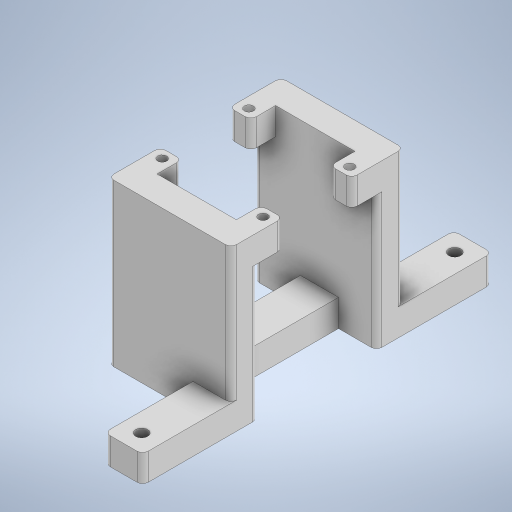
# Autodesk Inventor part: lepton mount
Saved by Autodesk Inventor 2024 (Build 280153000, 153)
## iProperties
Created: 2024-01-12
Part Number: lepton mount
Material: Generic
Document SubType Name: Modeling
Designer: Eli
Density: 1 g/cm^3
Appearance: Default
Author: Eli
Autodesk Inventor part; units mm, degrees
ref_plane "YZ Plane" through (0, 0, 0) normal (1, 0, 0) x (0, 1, 0)
ref_plane "XZ Plane" through (0, 0, 0) normal (0, 1, 0) x (-1, 0, 0)
ref_plane "XY Plane" through (0, 0, 0) normal (0, 0, 1) x (1, 0, 0)
sketch "Sketch1" plane through (0, 0, 0) normal (0, 1, 0) x (-1, 0, 0)
  line L0 (0, 0) -> (-8.9535, 0)
  line L1 (-8.9535, 0) -> (-8.9535, -82.296)
  line L2 (-8.9535, -82.296) -> (0, -82.296)
  line L3 (0, -82.296) -> (0, 0)
  circle A0 centre (-4.4767, -4.2545) radius 1.4224
  line L4 (0, -41.148) -> (-8.9535, -41.148) construction
  circle A1 centre (-4.4767, -78.0415) radius 1.4224
  line L5 (0, -20.828) -> (19.9009, -20.828)
  line L6 (19.9009, -20.828) -> (19.9009, -61.468)
  line L7 (19.9009, -61.468) -> (0, -61.468)
  line L8 (0, -61.468) -> (0, -20.828)
  line L9 (19.9009, -55.118) -> (0, -55.118)
  line L10 (0, -55.118) -> (0, -27.178)
  line L11 (0, -27.178) -> (19.9009, -27.178)
  line L12 (19.9009, -27.178) -> (19.9009, -55.118)
  line L13 (0, -55.118) -> (8.9662, -55.118)
  line L14 (8.9662, -55.118) -> (8.9662, -27.178)
  line L15 (8.9662, -27.178) -> (0, -27.178)
  line L16 (0, -27.178) -> (0, -55.118)
  line L17 (0, -27.178) -> (-8.9535, -27.178)
  line L18 (0, -55.118) -> (-8.9535, -55.118)
  line L19 (0, -20.828) -> (-8.9535, -20.828)
  line L20 (0, -61.468) -> (-8.9535, -61.468)
  point P0 (-4.4768, 0)
  point P1 (0, -61.468)
  point P2 (0, -55.118)
  point P3 (19.9009, -27.178)
  point P4 (0, -55.118)
  point P5 (0, -61.468)
  dimension "d0" = 82.296
  dimension "d1" = 8.9535
  dimension "d2" = 2.8448
  dimension "d3" = 4.2545
  dimension "d4" = 4.4768
  dimension "d5" = 40.64
  dimension "d6" = 19.9009
  dimension "d11" = 27.94
  dimension "d28" = 8.9662
  constraints: 42 end point, 8 parallel, 8 perpendicular, 8 point on line, 4 horizontal, 3 midpoint, 2 centre point, 1 symmetric about line, 3 other
  measures "d0" distance of L0.end L1.end
  measures "d1" distance of L0.start L0.end
  measures "d2" diameter of A0
  measures "d3" distance of point (-4.477, 0) A0.centre
  measures "d4" distance from line of L3 A0.centre
  measures "d5" distance of L5.end L6.end
  measures "d6" distance between parallel lines of L8 L6
  measures "d11" distance between parallel lines of L11 L9
  measures "d28" distance between parallel lines of L8 L14
extrude "Extrusion1" add sketch "Sketch1" along normal blind 6.35 contours L3 L19 L1 L0 | L11 L14 L9 L3 | L3 L2 L1 L20
fillet "Fillet1" radius 1.27 4 edges at (8.9535, 3.175, 0) (0, 3.175, 0) (8.9535, 3.175, -82.296) (0, 3.175, -82.296)
extrude "Extrusion2" add sketch "Sketch1" along normal blind 38.1 contours L5 L6 L11 L3 | L3 L17 L1 L19 | L9 L6 L7 L3 | L3 L20 L1 L18
sketch "Sketch2" plane through (-19.9009, 0, -55.118) normal (0, 0, 1) x (1, 0, 0)
  line L0 (0, 38.1) -> (19.9009, 38.1) projected
  line L1 (19.9009, 38.1) -> (23.7744, 38.1)
  line L2 (23.7744, 38.1) -> (23.7744, 31.75)
  line L3 (23.7744, 31.75) -> (28.8544, 31.75)
  line L4 (28.8544, 31.75) -> (28.8544, 38.1)
  line L5 (28.8544, 0) -> (28.8544, 38.1) projected
  line L6 (23.7744, 38.1) -> (28.8544, 38.1)
  line L7 (28.8544, 38.1) -> (28.8544, 31.75)
  point P0 (19.9009, 0)
  point P1 (14.8209, 38.1)
  dimension "d14" = 6.35
  dimension "d15" = 5.08
  constraints: 12 end point, 2 parallel, 2 perpendicular, 1 collinear, 1 horizontal
  measures "d14" distance of L1.end L2.end
  measures "d15" distance of L2.end L3.end
extrude "Extrusion3" add sketch "Sketch2" along normal blind 5.842
sketch "Sketch3" plane through (0, 38.1, 0) normal (0, 1, 0) x (1, 0, 0)
  line L0 (-19.9009, 55.118) -> (-8.9662, 55.118) construction
  line L1 (3.8735, 49.276) -> (8.9535, 49.276) construction
  line L2 (6.4135, 49.276) -> (6.4135, 55.118) construction
  line L3 (0, 55.118) -> (8.9535, 55.118) construction
  point P0 (0, 0)
  point P1 (6.4135, 51.3715)
  dimension "d34" = 2.0955
  dimension "d35" = 0
  constraints: 2 end point, 1 midpoint, 1 point on line, 1 vertical
  measures "d34" distance from line of L1 point (6.413, 51.371)
  measures "d35" distance from line of L2 point (6.413, 51.371)
hole "Hole1" at (6.4135, 38.1, -51.3715) direction (0, -1, 0) diameter 2.1463 depth 6.35 tip angle 118
ref_plane "Work Plane1" through (-5.4737, 0, -81.026) normal (1, 0, 0) x (0, 0, -1)
mirror "Mirror1" about plane through (-5.4737, 0, -81.026) normal (1, 0, 0) of "Extrusion3", "Hole1"
ref_plane "Work Plane2" through (-19.9009, 0, -41.148) normal (0, 0, 1) x (1, 0, 0)
mirror "Mirror2" about plane through (-19.9009, 0, -41.148) normal (0, 0, 1) of "Extrusion3", "Hole1", "Mirror1"
fillet "Fillet2" radius 1.27 2 edges at (-19.9009, 19.05, -20.828) (-19.9009, 19.05, -61.468)
fillet "Fillet3" radius 1.27 8 edges at (8.9535, 34.925, -49.276) (3.8735, 34.925, -49.276) (-14.8209, 34.925, -49.276) (-19.9009, 34.925, -49.276) (-19.9009, 34.925, -33.02) (3.8735, 34.925, -33.02) (-14.8209, 34.925, -33.02) (8.9535, 34.925, -33.02)
fillet "Fillet5" radius 1.27 2 edges at (-19.9009, 15.875, -55.118) (-19.9009, 15.875, -27.178)
fillet "Fillet7" radius 1.27 2 edges at (8.9535, 15.875, -27.178) (8.9535, 15.875, -55.118)
fillet "Fillet10" radius 1.27 2 edges at (8.9535, 22.225, -20.828) (8.9535, 22.225, -61.468)
body "Solid1"
